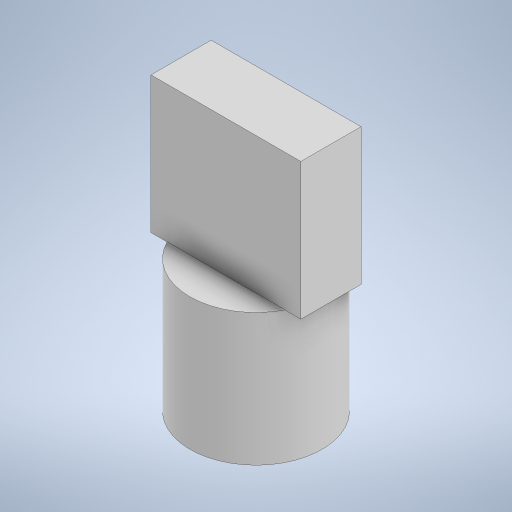
# Autodesk Inventor part: bone_attachment_3mm_test
Saved by Autodesk Inventor 2024 (Build 280153000, 153)
## iProperties
Created: 2024-06-07
Part Number: bone_attachment_3mm_test
Material: 일반
Document SubType Name: Modeling
Designer: Gihyeok Na
Density: 1 g/cm^3
Appearance: 기본값
Author: Gihyeok Na
Autodesk Inventor part; units mm, degrees
ref_plane "YZ Plane" through (0, 0, 0) normal (1, 0, 0) x (0, 1, 0)
ref_plane "XZ Plane" through (0, 0, 0) normal (0, 1, 0) x (-1, 0, 0)
ref_plane "XY Plane" through (0, 0, 0) normal (0, 0, 1) x (1, 0, 0)
sketch "스케치2" plane through (0, 0, 0) normal (0, 1, 0) x (-1, 0, 0)
  circle A0 centre (0, 0) radius 1.5
  dimension "d0" = 3
  constraints: 1 centre point, 1 coincident
  measures "d0" diameter of A0
extrude "돌출1" add sketch "스케치2" along normal blind 3
sketch "스케치3" plane through (0, 3, 0) normal (0, 1, 0) x (1, 0, 0)
  line L0 (1.7, -0.6824) -> (-1.7, -0.6824)
  line L1 (-1.7, -0.6824) -> (-1.7, 0.6824)
  line L2 (-1.7, 0.6824) -> (1.7, 0.6824)
  line L3 (1.7, 0.6824) -> (1.7, -0.6824)
  line L4 (1.7, -0.6824) -> (-1.7, 0.6824) construction
  line L5 (-1.7, -0.6824) -> (1.7, 0.6824) construction
  point P0 (0, 0)
  dimension "d3" = 3.4
  constraints: 12 end point, 2 midpoint, 2 parallel, 1 horizontal, 1 perpendicular
  measures "d3" distance of L1.end L2.end
extrude "돌출2" add sketch "스케치3" along normal blind 3.1
